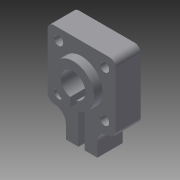
# Autodesk Inventor part: widget
Saved by Autodesk Inventor 2014 (Build 180170000, 170)
## iProperties
Created: 2013-07-24
Part Number: widget
Material: Generic
Document SubType Name: Modeling
Designer: Admin
Density: 1 g/cm^3
Appearance: Default
Author: Admin
Autodesk Inventor part; units mm, degrees
ref_plane "YZ Plane" through (0, 0, 0) normal (1, 0, 0) x (0, 1, 0)
ref_plane "XZ Plane" through (0, 0, 0) normal (0, 1, 0) x (-1, 0, 0)
ref_plane "XY Plane" through (0, 0, 0) normal (0, 0, 1) x (1, 0, 0)
sketch "Sketch1" plane through (0, 0, 0) normal (0, 0, 1) x (1, 0, 0)
  circle A0 centre (0, 0) radius 3.675
  circle A1 centre (0, 0) radius 6.35
  line L0 (-10.287, 10.287) -> (10.287, 10.287)
  line L1 (10.287, 10.287) -> (10.287, -10.287)
  line L2 (-10.287, -10.287) -> (-10.287, 10.287)
  line L3 (10.287, 10.287) -> (0, 10.287) construction
  circle A2 centre (-6.9596, 6.9596) radius 1.3716
  line L4 (-6.9596, 6.9596) -> (-10.287, 10.287) construction
  circle A3 centre (6.9596, 6.9596) radius 1.3716
  line L5 (6.9596, 6.9596) -> (10.287, 10.287) construction
  line L6 (-6.9596, 6.9596) -> (6.9596, 6.9596) construction
  circle A4 centre (-6.9596, -6.9596) radius 1.3716
  circle A5 centre (6.9596, -6.9596) radius 1.3716
  line L7 (-6.9596, 6.9596) -> (-6.9596, -6.9596) construction
  line L8 (-10.287, -10.287) -> (-8.2403, -10.287)
  line L9 (10.287, -10.287) -> (8.2403, -10.287)
  line L10 (21.5842, 10.287) -> (21.5842, 0) construction
  line L11 (21.5842, 0) -> (21.5842, -10.287) construction
  arc A6 (-4.7625, -13.7648) -> (-8.2403, -10.287) centre (-8.2403, -13.7648) ccw
  arc A7 (8.2403, -10.287) -> (4.7625, -13.7648) centre (8.2403, -13.7648) ccw
  line L12 (-4.7625, -13.7648) -> (-4.7625, -17.8424)
  line L13 (4.7625, -13.7648) -> (4.7625, -17.8424)
  line L14 (-4.7625, -17.8424) -> (4.7625, -17.8424)
  line L15 (0, -17.1877) -> (-4.7625, -17.1877) construction
  line L16 (0, -17.1877) -> (4.7625, -17.1877) construction
  point P0 (0, 10.287)
  dimension "d7" = 7.35
  dimension "d8" = 12.7
  dimension "d11" = 10.287
  dimension "d14" = 20.574
  dimension "d15" = 2.7432
  dimension "d16" = 45
  dimension "d18" = 2.7432
  dimension "d19" = 45
  dimension "d20" = 13.9192
  dimension "d21" = 2.7432
  dimension "d22" = 2.7432
  dimension "d23" = 13.9192
  dimension "d25" = 20.574
  dimension "d27" = 20.574
  dimension "d28" = 10.287
  dimension "d34" = 9.525
  dimension "d44" = 4.7625
  constraints: 34 end point, 8 centre point, 7 horizontal alignment, 6 perpendicular, 6 vertical alignment, 5 equal length, 4 point on circle, 3 tangent, 2 coincident, 2 point on line, 1 horizontal, 1 midpoint
  measures "d7" diameter of A0
  measures "d8" diameter of A1
  measures "d11" distance of L0.end L3.end
  measures "d14" distance of L0.end L1.end
  measures "d15" diameter of A2
  measures "d16" angle of L4 L2
  measures "d18" diameter of A3
  measures "d19" angle of L5 L1
  measures "d20" distance of L4.start L5.start
  measures "d21" diameter of A4
  measures "d22" diameter of A5
  measures "d23" distance of L4.start L7.end
  measures "d25" distance of L2.start L0.start
  measures "d27" distance of L0.start L0.end
  measures "d28" distance of L10.start L10.end
  measures "d34" distance of L12.end L13.end
  measures "d44" distance of L15.start L15.end
extrude "Extrusion1" add sketch "Sketch1" along normal blind 7.62 contours A1 | L0 L1 L9 A7 L13 L14 L12 A6 L8 L2
sketch "Sketch2" plane through (0, 0, 7.62) normal (0, 0, 1) x (1, 0, 0)
  circle A0 centre (0, 0) radius 3.675 projected
  circle A1 centre (0, 0) radius 6.35
  dimension "d37" = 12.7
  constraints: 1 centre point, 1 coincident
  measures "d37" diameter of A1
extrude "Extrusion2" add sketch "Sketch2" along normal blind 2.54
fillet "Fillet1" radius 1.905 1 edges at (10.287, 10.287, 3.81)
fillet "Fillet2" radius 1.905 1 edges at (-10.287, 10.287, 3.81)
fillet "Fillet3" radius 1.905 1 edges at (-10.287, -10.287, 3.81)
fillet "Fillet4" radius 1.905 1 edges at (10.287, -10.287, 3.81)
sketch "Sketch3" plane through (0, 0, 0) normal (0, 0, -1) x (-1, 0, 0)
  line L0 (-4.7625, -13.7648) -> (-4.7625, -17.8424) projected
  line L1 (-4.7625, -17.8424) -> (4.7625, -17.8424) projected
  line L2 (4.7625, -17.8424) -> (4.7625, -13.7648) projected
  line L3 (-10.287, 8.382) -> (-10.287, -8.382) projected
  circle A0 centre (0, 0) radius 3.675 projected
  line L4 (-4.7625, -17.8424) -> (-0.9525, -17.8424) construction
  line L5 (4.7625, -16.7338) -> (0.9525, -16.7338) construction
  line L6 (-0.9525, -17.8424) -> (-0.9525, -3.5494)
  line L7 (0.9525, -17.8424) -> (0.9525, -3.5494)
  line L8 (-0.9525, -17.8424) -> (0.9525, -17.8424)
  arc A1 (-0.9525, -3.5494) -> (0.9525, -3.5494) centre (0, 0) ccw
  dimension "d45" = 3.81
  dimension "d46" = 3.81
  constraints: 10 end point, 4 point on circle, 4 point on line, 3 perpendicular, 2 parallel, 1 centre point, 1 collinear, 1 concentric
  measures "d45" distance of L4.start L4.end
  measures "d46" distance of L5.start L5.end
extrude "Extrusion3" cut sketch "Sketch3" against normal blind 10.16 contours L6 A0 L7 L1
equation "\"d11\" = 0.5 * d9"
equation "\"d14\" = d9"
equation "\"d18\" = d15"
equation "\"d19\" = d16"
equation "\"d21\" = d15"
equation "\"d22\" = d15"
equation "\"d23\" = d20"
equation "\"d25\" = d14"
equation "\"d27\" = d25"
equation "\"d28\" = 0.5 * d14"
equation "\"d44\" = 0.5 * d34"
equation "\"d46\" = d45"
equation "\"d9\" = 20.574"
body "Solid1"
